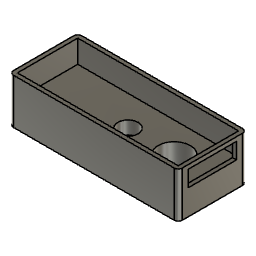
Support_LeapMotion (Autodesk Fusion 360 design; units mm, degrees)
Autodesk Fusion 360 part; units mm, degrees
note: some values were not read from the file. Chosen so that the rebuilt part matches the saved one: which face or edge a step refers to.
sketch "Esquisse1" plane through (0, 0, 0) normal (0, 0, 1) x (1, 0, 0)
  line L0 (0, 0) -> (84, 0)
  line L1 (84, 0) -> (84, 34)
  line L2 (84, 34) -> (0, 34)
  line L3 (0, 34) -> (0, 0)
  dimension "d1" = 34
  dimension "d2" = 84
  constraint horizontal L0
  constraint vertical L1
  constraint horizontal L2
  constraint vertical L3
  constraint coincident L0.start L3.end
  measures "d1" distance of L0 L2
  measures "d2" distance of L1 L3
extrude "Extrusion1" add sketch "Esquisse1" along normal blind 14
sketch "Esquisse2" plane through (0, 0, 14) normal (0, 0, 1) x (-1, 0, 0)
  line L0 (0, -34) -> (0, 0)
  line L1 (0, 0) -> (-84, 0)
  line L2 (-84, 0) -> (-84, -34)
  line L3 (-84, -34) -> (0, -34)
  line L4 (-2, -32) -> (-82, -32)
  line L5 (-82, -32) -> (-82, -2)
  line L6 (-82, -2) -> (-2, -2)
  line L7 (-2, -2) -> (-2, -32)
  dimension "d5" = 2
  dimension "d6" = 2
  dimension "d7" = 2
  dimension "d8" = 2
  constraint horizontal L4
  constraint vertical L5
  constraint horizontal L6
  constraint vertical L7
  measures "d5" distance of L0 L7
  measures "d6" distance of L2 L5
  measures "d7" distance of L3 L4
  measures "d8" distance of L1 L6
extrude "Extrusion2" cut sketch "Esquisse2" against normal blind 11.3 contours L4 L5 L6 L7
sketch "Esquisse3" plane through (84, 0, 0) normal (1, 0, 0) x (0, 1, 0)
  line L0 (0, 0) -> (34, 0)
  line L1 (34, 0) -> (34, 14)
  line L2 (34, 14) -> (0, 14)
  line L3 (0, 14) -> (0, 0)
  line L4 (5, 12) -> (29, 12)
  line L5 (29, 12) -> (29, 4)
  line L6 (29, 4) -> (5, 4)
  line L7 (5, 4) -> (5, 12)
  dimension "d12" = 2
  dimension "d13" = 8
  dimension "d14" = 5
  dimension "d15" = 5
  constraint horizontal L4
  constraint vertical L5
  constraint horizontal L6
  constraint vertical L7
  measures "d12" distance of L2 L4
  measures "d13" distance of L4 L6
  measures "d14" distance of L3 L7
  measures "d15" distance of L1 L5
extrude "Extrusion6" add 1 faces at (28, 22.6667, 0) along direction (0, 0, -1) blind 6.5
sketch "Esquisse6" plane through (0, 0, 2.7) normal (0, 0, 1) x (-1, 0, 0)
  line L0 (-2, -2) -> (-82, -2)
  line L1 (-82, -2) -> (-82, -32)
  line L2 (-82, -32) -> (-2, -32)
  line L3 (-2, -32) -> (-2, -2)
  circle A0 centre (-42, -17) radius 5
  dimension "d26" = 10
  dimension "d27" = 15
  dimension "d30" = 40
  measures "d26" diameter of A0
  measures "d27" distance of L2 A0.centre
  measures "d30" distance of L3 A0.centre
extrude "Extrusion7" cut sketch "Esquisse6" against normal blind 6.5 contours A0
sketch "Esquisse7" plane through (0, 0, -6.5) normal (0, 0, -1) x (1, 0, 0)
  line L0 (0, 0) -> (0, -34)
  line L1 (0, -34) -> (84, -34)
  line L2 (84, -34) -> (84, 0)
  line L3 (84, 0) -> (0, 0)
  circle A0 centre (42, -17) radius 3.25
  dimension "d31" = 6.5
  dimension "d32" = 42
  measures "d31" diameter of A0
  measures "d32" distance of L0 A0.centre
extrude "Extrusion8" cut sketch "Esquisse7" against normal blind 10 contours A0
extrude "Extrusion9" cut sketch "Esquisse3" against normal blind 8 contours L4 L5 L6 L7
sketch "Esquisse8" plane through (0, 0, 14) normal (0, 0, 1) x (-1, 0, 0)
  circle A0 centre (-65, -17) radius 8
  dimension "d37" = 16
  measures "d37" diameter of A0
extrude "Extrusion10" cut sketch "Esquisse8" against normal blind 43
fillet "Congé1" radius 2 1 edges at (84, 0, 3.75)
fillet "Congé2" radius 2 1 edges at (84, 34, 3.75)
fillet "Congé3" radius 2 1 edges at (0, 34, 3.75)
fillet "Congé4" radius 2 1 edges at (0, 0, 3.75)
extrude "Extrusion11" add sketch "Esquisse7" along normal blind 3
fillet "Congé5" radius 2 1 edges at (0, 0, -8)
fillet "Congé6" radius 2 1 edges at (0, 34, -8)
fillet "Congé7" radius 2 1 edges at (84, 34, -8)
fillet "Congé8" radius 2 1 edges at (84, 0, -8)
extrude "Extrusion12" cut 1 faces at (12.9167, 17, -9.5) along direction (0, 0, 1) blind 1
extrude "Extrusion13" cut 1 faces at (67.2837, 16.3989, -6.5) along direction (0, 0, -1) blind 10
extrude "Extrusion3" [suppressed]
sketch "Esquisse5" plane through (0, 0, 0) normal (0, 0, -1) x (1, 0, 0)
  line L0 (0, 0) -> (0, -34)
  line L1 (0, -34) -> (84, -34)
  line L2 (84, -34) -> (84, 0)
  line L3 (84, 0) -> (0, 0)
  circle A0 centre (20, -18) radius 10
  dimension "d18" = 18
  dimension "d19" = 20
  measures "d18" distance of L3 A0.centre
  measures "d19" diameter of A0
extrude "Extrusion4" [suppressed]
extrude "Extrusion5" [suppressed]
equation "d20 = -( 14 mm - 11.3 mm )"
